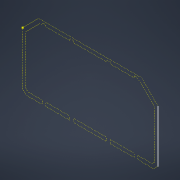
# Autodesk Inventor part: PlanchaBaseInferior
Saved by Autodesk Inventor 2022 (Build 260153000, 153)
## iProperties
Created: 2021-09-22
Part Number: PlanchaBaseInferior
Material: Steel, Mild, Welded
Document SubType Name: Sheet Metal
Designer: Andres
Density: 7.85 g/cm^3
Sheet Metal Rule: Default_mm
Appearance: Weld - Steel Mild
Author: Andres
Autodesk Inventor part; units mm, degrees
ref_plane "YZ Plane" through (0, 0, 0) normal (1, 0, 0) x (0, 1, 0)
ref_plane "XZ Plane" through (0, 0, 0) normal (0, 1, 0) x (-1, 0, 0)
ref_plane "XY Plane" through (0, 0, 0) normal (0, 0, 1) x (1, 0, 0)
sketch "Sketch1" plane through (0, 0, 0) normal (0, 0, 1) x (1, 0, 0)
  line L0 (126.4853, -370.4853) -> (126.4853, -346.4853) construction
  line L1 (126.4853, -346.4853) -> (33.4558, -346.4853) construction
  line L2 (33.4558, -346.4853) -> (20.4853, -333.5147) construction
  line L3 (20.4853, -333.5147) -> (20.4853, -13.4558) construction
  line L4 (20.4853, -13.4558) -> (113.4558, 79.5147) construction
  line L5 (113.4558, 79.5147) -> (126.4853, 79.5147) construction
  line L6 (126.4853, 79.5147) -> (126.4853, 91.5147) construction
  line L7 (126.4853, 91.5147) -> (150.4853, 91.5147) construction
  line L8 (150.4853, 79.5147) -> (150.4853, 91.5147) construction
  line L9 (150.4853, 79.5147) -> (306.4853, 79.5147) construction
  line L10 (306.4853, 91.5147) -> (306.4853, 79.5147) construction
  line L11 (306.4853, 91.5147) -> (330.4853, 91.5147) construction
  line L12 (330.4853, 91.5147) -> (330.4853, 79.5147) construction
  line L13 (330.4853, 79.5147) -> (546.4853, 79.5147) construction
  line L14 (546.4853, 91.5147) -> (546.4853, 79.5147) construction
  line L15 (546.4853, 91.5147) -> (570.4853, 91.5147) construction
  line L16 (570.4853, 91.5147) -> (570.4853, 79.5147) construction
  line L17 (570.4853, 79.5147) -> (726.4853, 79.5147) construction
  line L18 (726.4853, 79.5147) -> (726.4853, 91.5147) construction
  line L19 (726.4853, 91.5147) -> (750.4853, 91.5147) construction
  line L20 (750.4853, 79.5147) -> (750.4853, 91.5147) construction
  line L21 (750.4853, 79.5147) -> (763.5147, 79.5147) construction
  line L22 (763.5147, 79.5147) -> (856.4853, -13.4558) construction
  line L23 (856.4853, -13.4558) -> (856.4853, -333.5147) construction
  line L24 (856.4853, -333.5147) -> (843.5147, -346.4853) construction
  line L25 (843.5147, -346.4853) -> (750.4853, -346.4853) construction
  line L26 (750.4853, -370.4853) -> (750.4853, -346.4853) construction
  line L27 (853.4558, -370.4853) -> (750.4853, -370.4853) construction
  line L28 (880.4853, -343.4558) -> (853.4558, -370.4853) construction
  line L29 (880.4853, -3.5147) -> (880.4853, -343.4558) construction
  line L30 (773.4558, 103.5147) -> (880.4853, -3.5147) construction
  line L31 (103.5147, 103.5147) -> (773.4558, 103.5147) construction
  line L32 (-3.5147, -3.5147) -> (103.5147, 103.5147) construction
  line L33 (-3.5147, -343.4558) -> (-3.5147, -3.5147) construction
  line L34 (23.5147, -370.4853) -> (-3.5147, -343.4558) construction
  line L35 (126.4853, -370.4853) -> (23.5147, -370.4853) construction
  line L36 (330.4853, -346.4853) -> (330.4853, -370.4853) construction
  line L37 (546.4853, -370.4853) -> (330.4853, -370.4853) construction
  line L38 (546.4853, -346.4853) -> (546.4853, -370.4853) construction
  line L39 (546.4853, -346.4853) -> (330.4853, -346.4853) construction
  line L40 (726.4853, -370.4853) -> (726.4853, -346.4853) construction
  line L41 (726.4853, -346.4853) -> (570.4853, -346.4853) construction
  line L42 (570.4853, -346.4853) -> (570.4853, -370.4853) construction
  line L43 (726.4853, -370.4853) -> (570.4853, -370.4853) construction
  line L44 (150.4853, -370.4853) -> (150.4853, -346.4853) construction
  line L45 (306.4853, -370.4853) -> (150.4853, -370.4853) construction
  line L46 (306.4853, -346.4853) -> (306.4853, -370.4853) construction
  line L47 (306.4853, -346.4853) -> (150.4853, -346.4853) construction
  line L48 (880.4853, -3.5147) -> (880.4853, -343.4558)
  line L49 (853.4558, -370.4853) -> (23.5147, -370.4853)
  line L50 (23.5147, -370.4853) -> (-3.5147, -343.4558)
  line L51 (-3.5147, -343.4558) -> (-3.5147, -3.5147)
  line L52 (-3.5147, -3.5147) -> (103.5147, 103.5147)
  line L53 (103.5147, 103.5147) -> (773.4558, 103.5147)
  line L54 (773.4558, 103.5147) -> (880.4853, -3.5147)
  line L55 (880.4853, -343.4558) -> (853.4558, -370.4853)
  point P0 (0, 0)
extrude "Plate1" add sketch "Sketch1" along normal blind 0.5
sketch "Sketch2" plane through (0, 0, 0.5) normal (0, 0, 1) x (1, 0, 0)
  line L0 (118.4853, -25.4853) -> (38.4853, -25.4853)
  line L1 (38.4853, -25.4853) -> (38.4853, -325.4853)
  line L2 (38.4853, -325.4853) -> (118.4853, -325.4853)
  line L3 (118.4853, -325.4853) -> (118.4853, -25.4853)
  line L4 (118.4853, -25.4853) -> (38.4853, -325.4853) construction
  line L5 (38.4853, -25.4853) -> (118.4853, -325.4853) construction
  line L6 (119.5571, -346.4853) -> (119.5571, -370.4853) projected
  line L7 (119.5571, -370.4853) -> (23.5147, -370.4853) projected
  line L8 (23.5147, -370.4853) -> (-3.5147, -343.4558) projected
  line L9 (-3.5147, -343.4558) -> (-3.5147, -3.5147) projected
  line L10 (-3.5147, -3.5147) -> (103.5147, 103.5147) projected
  line L11 (103.5147, 103.5147) -> (773.4558, 103.5147) projected
  line L12 (773.4558, 103.5147) -> (880.4853, -3.5147) projected
  line L13 (880.4853, -3.5147) -> (880.4853, -343.4558) projected
  line L14 (880.4853, -343.4558) -> (853.4558, -370.4853) projected
  line L15 (853.4558, -370.4853) -> (757.4135, -370.4853) projected
  line L16 (757.4135, -370.4853) -> (757.4135, -346.4853) projected
  line L17 (843.5147, -346.4853) -> (757.4135, -346.4853) projected
  line L18 (856.4853, -333.5147) -> (843.5147, -346.4853) projected
  line L19 (856.4853, -13.4558) -> (856.4853, -333.5147) projected
  line L20 (763.5147, 79.5147) -> (856.4853, -13.4558) projected
  line L21 (757.4135, 79.5147) -> (763.5147, 79.5147) projected
  line L22 (757.4135, 79.5147) -> (757.4135, 91.5147) projected
  line L23 (757.4135, 91.5147) -> (719.5571, 91.5147) projected
  line L24 (719.5571, 91.5147) -> (719.5571, 79.5147) projected
  line L25 (577.4135, 79.5147) -> (719.5571, 79.5147) projected
  line L26 (577.4135, 79.5147) -> (577.4135, 91.5147) projected
  line L27 (577.4135, 91.5147) -> (539.5571, 91.5147) projected
  line L28 (539.5571, 91.5147) -> (539.5571, 79.5147) projected
  line L29 (337.4135, 79.5147) -> (539.5571, 79.5147) projected
  line L30 (337.4135, 79.5147) -> (337.4135, 91.5147) projected
  line L31 (337.4135, 91.5147) -> (299.5571, 91.5147) projected
  line L32 (299.5571, 91.5147) -> (299.5571, 79.5147) projected
  line L33 (157.4135, 79.5147) -> (299.5571, 79.5147) projected
  line L34 (157.4135, 79.5147) -> (157.4135, 91.5147) projected
  line L35 (157.4135, 91.5147) -> (119.5571, 91.5147) projected
  line L36 (119.5571, 91.5147) -> (119.5571, 79.5147) projected
  line L37 (113.4558, 79.5147) -> (119.5571, 79.5147) projected
  line L38 (20.4853, -13.4558) -> (113.4558, 79.5147) projected
  line L39 (20.4853, -333.5147) -> (20.4853, -13.4558) projected
  line L40 (33.4558, -346.4853) -> (20.4853, -333.5147) projected
  line L41 (119.5571, -346.4853) -> (33.4558, -346.4853) projected
  line L42 (438.4853, 188.8971) -> (438.4853, -449.5258) construction
  line L43 (758.4853, -25.4853) -> (838.4853, -25.4853)
  line L44 (838.4853, -25.4853) -> (838.4853, -325.4853)
  line L45 (838.4853, -325.4853) -> (758.4853, -325.4853)
  line L46 (758.4853, -325.4853) -> (758.4853, -25.4853)
  line L47 (758.4853, -25.4853) -> (838.4853, -325.4853) construction
  line L48 (838.4853, -25.4853) -> (758.4853, -325.4853) construction
  point P0 (0, 0)
  point P1 (78.4853, -175.4853)
  point P2 (438.4853, 79.5147)
  point P3 (798.4853, -175.4853)
  dimension "d1" = 80
  dimension "d2" = 300
  dimension "d4" = 360
  dimension "d5" = 255
  constraints: 26 end point, 5 midpoint, 5 symmetric about line, 2 parallel, 1 horizontal, 1 perpendicular, 1 vertical, 1 vertical alignment
  measures "d1" distance between parallel lines of L1 L3
  measures "d2" distance between parallel lines of L2 L0
  measures "d4" distance from line of point (78.485, -175.485) L42
  measures "d5" vertical distance of point (438.485, 79.515) point (78.485, -175.485)
extrude "Cut1" cut sketch "Sketch2" against normal through all contours L3 L2 L1 L0 | L43 L44 L45 L46
fillet "Corner Round1" radius 6 8 edges at (118.4853, -25.4853, 0.25) (38.4853, -25.4853, 0.25) (38.4853, -325.4853, 0.25) (118.4853, -325.4853, 0.25) (838.4853, -25.4853, 0.25) (758.4853, -25.4853, 0.25) (838.4853, -325.4853, 0.25) (758.4853, -325.4853, 0.25)
equation "\"d6\" = Thickness"
equation "\"d0\" = Thickness"
equation "\"BendRadius\" = Thickness"
equation "\"BendReliefWidth\" = Thickness"
equation "\"BendReliefDepth\" = 0.5 * Thickness"
equation "\"CornerReliefSize\" = 4 * Thickness"
equation "\"MinimumRemnant\" = 2 * Thickness"
equation "\"TransitionRadius\" = BendRadius"
equation "\"JacobiRadiusSize\" = BendRadius"
equation "\"GapSize\" = Thickness"
equation "\"Thickness\" = 0.5"
body "Solid1"
